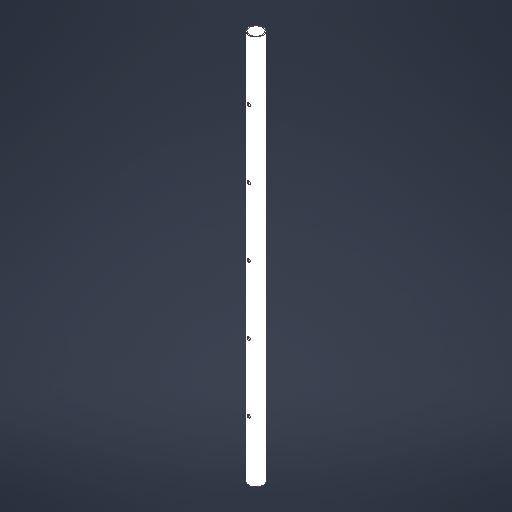
# Autodesk Inventor part: Pieza37
Saved by Autodesk Inventor 2026.2 (Build 302298000, 298)
## iProperties
Created: 2026-01-02
Part Number: Pieza37
Material: Genérico
Document SubType Name: Modeling
Designer: vicho
Density: 1 g/cm^3
Appearance: Valor por defecto
Author: vicho
Autodesk Inventor part; units mm, degrees
ref_plane "YZ Plane" through (0, 0, 0) normal (1, 0, 0) x (0, 1, 0)
ref_plane "XZ Plane" through (0, 0, 0) normal (0, 1, 0) x (-1, 0, 0)
sketch "Boceto1" plane through (0, 0, 0) normal (0, 1, 0) x (-1, 0, 0)
  circle A0 centre (0, 0) radius 17.5
  dimension "d0" = 35
  constraints: 1 centre point, 1 coincident
  measures "d0" diameter of A0
extrude "Extrusión1" add sketch "Boceto1" along normal blind 925
shell "Vaciado1" thickness 2 removed faces 2 at (-4.865, 0, -5.1831) at (-4.865, 925, -5.1831)
ref_plane "Plano de trabajo1" through (0, 0, 17.5) normal (0, 0, 1) x (1, 0, 0)
sketch "Boceto2" plane through (0, 0, 17.5) normal (0, 0, 1) x (1, 0, 0)
  line L0 (0, 994.5794) -> (0, -115.4582) construction
  line L1 (-550.5031, 0) -> (592.7318, 0) construction
  circle A0 centre (0, 782) radius 4
  line L2 (17.5, 925) -> (-17.5, 925) projected
  circle A1 centre (0, 622) radius 4
  circle A2 centre (0, 462) radius 4
  circle A3 centre (0, 302) radius 4
  circle A4 centre (0, 142) radius 4
  point P0 (0, 0)
  dimension "d5" = 8
  dimension "d6" = 143
  dimension "d7" = 8
  dimension "d8" = 8
  dimension "d9" = 8
  dimension "d10" = 8
  dimension "d11" = 160
  dimension "d12" = 160
  dimension "d13" = 160
  dimension "d14" = 160
  constraints: 7 point on line, 5 centre point, 4 end point, 1 horizontal, 1 vertical
  measures "d5" diameter of A0
  measures "d6" distance from line of L2 A0.centre
  measures "d7" diameter of A1
  measures "d8" diameter of A2
  measures "d9" diameter of A3
  measures "d10" diameter of A4
  measures "d11" distance of A1.centre A0.centre
  measures "d12" distance of A1.centre A2.centre
  measures "d13" distance of A2.centre A3.centre
  measures "d14" distance of A3.centre A4.centre
extrude "Extrusión2" cut sketch "Boceto2" against normal blind 50
